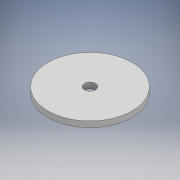
# Autodesk Inventor part: Aimant_tenir
Saved by Autodesk Inventor 2017 (Build 210142000, 142)
## iProperties
Part Number: Aimant_tenir
Material: Générique
Document SubType Name: Modeling
Designer: Darren
Density: 1 g/cm^3
Appearance: Par défaut
Author: Darren
Autodesk Inventor part; units mm, degrees
ref_plane "YZ Plane" through (0, 0, 0) normal (1, 0, 0) x (0, 1, 0)
ref_plane "XZ Plane" through (0, 0, 0) normal (0, 1, 0) x (-1, 0, 0)
ref_plane "XY Plane" through (0, 0, 0) normal (0, 0, 1) x (1, 0, 0)
sketch "Esquisse1" plane through (0, 0, 0) normal (0, 0, 1) x (1, 0, 0)
  circle A0 centre (0, 0) radius 2.875
  circle A1 centre (0, 0) radius 21.75
  dimension "d0" = 5.75
  dimension "d1" = 43.5
  constraints: 2 centre point, 2 coincident
  measures "d0" diameter of A0
  measures "d1" diameter of A1
extrude "Extrusion1" add sketch "Esquisse1" along normal blind 3
